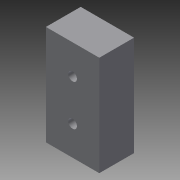
# Autodesk Inventor part: LDR_Shield
Saved by Autodesk Inventor 2015 SP2 (Build 190223200, 223)
## iProperties
Created: 2016-09-15
Part Number: LDR_Shield
Material: Generic
Document SubType Name: Modeling
Designer: jm799
Density: 1 g/cm^3
Appearance: Default
Author: jm799
Autodesk Inventor part; units mm, degrees
ref_plane "YZ Plane" through (0, 0, 0) normal (1, 0, 0) x (0, 1, 0)
ref_plane "XZ Plane" through (0, 0, 0) normal (0, 1, 0) x (-1, 0, 0)
ref_plane "XY Plane" through (0, 0, 0) normal (0, 0, 1) x (1, 0, 0)
sketch "Sketch1" plane through (0, 0, 0) normal (0, 1, 0) x (-1, 0, 0)
  line L0 (3.07, 5.7495) -> (-3.07, 5.7495)
  line L1 (-3.07, 5.7495) -> (-3.07, -5.7495)
  line L2 (-3.07, -5.7495) -> (3.07, -5.7495)
  line L3 (3.07, -5.7495) -> (3.07, 5.7495)
  line L4 (3.07, 0) -> (-3.07, 0) construction
  line L5 (0, 5.7495) -> (0, -5.7495) construction
  point P0 (0, 0)
  point P1 (0, 0)
  point P2 (0, 0)
  point P3 (0, 0)
  dimension "d0" = 6.14
  dimension "d1" = 11.499
  constraints: 12 end point, 5 midpoint, 3 coincident, 2 parallel, 1 horizontal, 1 perpendicular
  measures "d0" distance of L0.start L0.end
  measures "d1" distance of L0.end L1.end
extrude "Extrusion1" add sketch "Sketch1" along normal blind 4.001
sketch "Sketch2" plane through (0, 4.001, 0) normal (0, 1, 0) x (1, 0, 0)
  line L0 (-7.624, -4.7495) -> (2.376, -4.7495)
  line L1 (2.376, -4.7495) -> (2.376, 4.7495)
  line L2 (2.376, 4.7495) -> (-7.624, 4.7495)
  line L3 (-7.624, 4.7495) -> (-7.624, -4.7495)
  line L4 (-5, 0) -> (5, 0) construction
  line L5 (0, -4.7495) -> (0, 4.7495) construction
  point P0 (0, 0)
  point P1 (0, 0)
  point P2 (0, 0)
  dimension "d4" = 9.499
  dimension "d5" = 10
  constraints: 12 end point, 2 coincident, 2 midpoint, 2 parallel, 1 horizontal, 1 perpendicular
  measures "d4" distance of L0.end L1.end
  measures "d5" distance of L0.start L0.end
extrude "Extrusion2" cut sketch "Sketch2" against normal blind 3.001
sketch "Sketch3" plane through (0, 0, 0) normal (0, -1, 0) x (1, 0, 0)
  circle A0 centre (0, -2.356) radius 0.5
  line L0 (-3.07, 4.7495) -> (-3.07, -4.7495) construction
  line L1 (-3.07, 0) -> (3.07, 0) construction
  line L2 (3.07, 5.7495) -> (3.07, -5.7495) construction
  circle A1 centre (0, 2.356) radius 0.5
  point P0 (0, 0)
  dimension "d8" = 1
  constraints: 2 centre point, 2 end point, 2 midpoint, 1 symmetric about line, 1 other
  measures "d8" diameter of A0
hole "Hole1" at (0, 0, -2.356) at (0, 0, 2.356) direction (0, 1, 0) diameter 1 end through all
body "Solid1"
